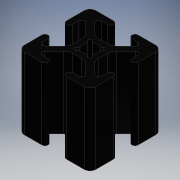
# Autodesk Inventor part: 1010-S-BLACK-FB
Saved by Autodesk Inventor 2017 SP1 (Build 210196100, 196)
## iProperties
Created: 2016-09-13
Part Number: 1010-S-BLACK-FB
Material: 6061-T6
Description: 40 S SHORT SINGLE UNIBEARING ASSEMBLY ON 40-4040 X 75mm
Document SubType Name: Modeling
Designer: BRALEF
Density: 1 g/cm^3
Appearance: BLACK ANODIZED
MATERIAL: 6061-T6
PART PRICE: 44.65
Author: BRALEF
Autodesk Inventor part; units mm, degrees
ref_plane "YZ Plane" through (0, 0, 0) normal (1, 0, 0) x (0, 1, 0)
ref_plane "XZ Plane" through (0, 0, 0) normal (0, 1, 0) x (-1, 0, 0)
ref_plane "XY Plane" through (0, 0, 0) normal (0, 0, 1) x (1, 0, 0)
sketch "Sketch1" plane through (0, 0, 0) normal (0, 1, 0) x (-1, 0, 0)
  arc A0 (-1.9692, 2.8605) -> (-2.8605, 1.9692) centre (-2.4696, 2.4696) ccw
  line L0 (-2.2319, 1.3405) -> (-2.8605, 1.9692)
  arc A1 (-2.2319, 1.3405) -> (-2.2319, -1.3405) centre (0, 0) ccw
  line L1 (-2.8605, -1.9692) -> (-2.2319, -1.3405)
  arc A2 (-2.8605, -1.9692) -> (-1.9692, -2.8605) centre (-2.4696, -2.4696) ccw
  line L2 (-1.3405, -2.2319) -> (-1.9692, -2.8605)
  arc A3 (-1.3405, -2.2319) -> (1.3405, -2.2319) centre (0, 0) ccw
  line L3 (1.9692, -2.8605) -> (1.3405, -2.2319)
  arc A4 (1.9692, -2.8605) -> (2.8605, -1.9692) centre (2.4696, -2.4696) ccw
  line L4 (2.2319, -1.3405) -> (2.8605, -1.9692)
  arc A5 (2.2319, -1.3405) -> (2.2319, 1.3405) centre (0, 0) ccw
  line L5 (2.8605, 1.9692) -> (2.2319, 1.3405)
  arc A6 (2.8605, 1.9692) -> (1.9692, 2.8605) centre (2.4696, 2.4696) ccw
  line L6 (1.3405, 2.2319) -> (1.9692, 2.8605)
  arc A7 (1.3405, 2.2319) -> (-1.3405, 2.2319) centre (0, 0) ccw
  line L7 (-1.9692, 2.8605) -> (-1.3405, 2.2319)
  arc A8 (-1.6396, -4.5172) -> (-3.8846, -5.4471) centre (-1.6396, -7.6922) ccw
  line L8 (-3.8846, -5.4471) -> (-7.1933, -8.7558)
  arc A9 (-7.1933, -8.7558) -> (-6.4749, -10.4902) centre (-6.4749, -9.4742) ccw
  line L9 (-6.4749, -10.4902) -> (-4.3561, -10.4902)
  arc A10 (-4.3561, -12.7) -> (-4.3561, -10.4902) centre (-4.3561, -11.5951) ccw
  line L10 (-4.3561, -12.7) -> (-10.5918, -12.7)
  arc A11 (-12.7, -10.5918) -> (-10.5918, -12.7) centre (-10.5918, -10.5918) ccw
  line L11 (-12.7, -10.5918) -> (-12.7, -4.3561)
  arc A12 (-10.4902, -4.3561) -> (-12.7, -4.3561) centre (-11.5951, -4.3561) ccw
  line L12 (-10.4902, -4.3561) -> (-10.4902, -6.4749)
  arc A13 (-10.4902, -6.4749) -> (-8.7558, -7.1933) centre (-9.4742, -6.4749) ccw
  line L13 (-8.7558, -7.1933) -> (-5.4471, -3.8846)
  arc A14 (-5.4471, -3.8846) -> (-4.5172, -1.6396) centre (-7.6922, -1.6396) ccw
  line L14 (-4.5172, -1.6396) -> (-4.5172, 1.6396)
  arc A15 (-4.5172, 1.6396) -> (-5.4471, 3.8846) centre (-7.6922, 1.6396) ccw
  line L15 (-5.4471, 3.8846) -> (-8.7558, 7.1933)
  arc A16 (-8.7558, 7.1933) -> (-10.4902, 6.4749) centre (-9.4742, 6.4749) ccw
  line L16 (-10.4902, 6.4749) -> (-10.4902, 4.3561)
  arc A17 (-12.7, 4.3561) -> (-10.4902, 4.3561) centre (-11.5951, 4.3561) ccw
  line L17 (-12.7, 4.3561) -> (-12.7, 10.5918)
  arc A18 (-10.5918, 12.7) -> (-12.7, 10.5918) centre (-10.5918, 10.5918) ccw
  line L18 (-10.5918, 12.7) -> (-4.3561, 12.7)
  arc A19 (-4.3561, 10.4902) -> (-4.3561, 12.7) centre (-4.3561, 11.5951) ccw
  line L19 (-4.3561, 10.4902) -> (-6.4749, 10.4902)
  arc A20 (-6.4749, 10.4902) -> (-7.1933, 8.7558) centre (-6.4749, 9.4742) ccw
  line L20 (-7.1933, 8.7558) -> (-3.8846, 5.4471)
  arc A21 (-3.8846, 5.4471) -> (-1.6396, 4.5172) centre (-1.6396, 7.6922) ccw
  line L21 (-1.6396, 4.5172) -> (1.6396, 4.5172)
  arc A22 (1.6396, 4.5172) -> (3.8846, 5.4471) centre (1.6396, 7.6922) ccw
  line L22 (3.8846, 5.4471) -> (7.1933, 8.7558)
  arc A23 (7.1933, 8.7558) -> (6.4749, 10.4902) centre (6.4749, 9.4742) ccw
  line L23 (6.4749, 10.4902) -> (4.3561, 10.4902)
  arc A24 (4.3561, 12.7) -> (4.3561, 10.4902) centre (4.3561, 11.5951) ccw
  line L24 (4.3561, 12.7) -> (10.5918, 12.7)
  arc A25 (12.7, 10.5918) -> (10.5918, 12.7) centre (10.5918, 10.5918) ccw
  line L25 (12.7, 10.5918) -> (12.7, 4.3561)
  arc A26 (10.4902, 4.3561) -> (12.7, 4.3561) centre (11.5951, 4.3561) ccw
  line L26 (10.4902, 4.3561) -> (10.4902, 6.4749)
  arc A27 (10.4902, 6.4749) -> (8.7558, 7.1933) centre (9.4742, 6.4749) ccw
  line L27 (8.7558, 7.1933) -> (5.4471, 3.8846)
  arc A28 (5.4471, 3.8846) -> (4.5172, 1.6396) centre (7.6922, 1.6396) ccw
  line L28 (4.5172, 1.6396) -> (4.5172, -1.6396)
  arc A29 (4.5172, -1.6396) -> (5.4471, -3.8846) centre (7.6922, -1.6396) ccw
  line L29 (5.4471, -3.8846) -> (8.7558, -7.1933)
  arc A30 (8.7558, -7.1933) -> (10.4902, -6.4749) centre (9.4742, -6.4749) ccw
  line L30 (10.4902, -6.4749) -> (10.4902, -4.3561)
  arc A31 (12.7, -4.3561) -> (10.4902, -4.3561) centre (11.5951, -4.3561) ccw
  line L31 (12.7, -4.3561) -> (12.7, -10.5918)
  arc A32 (10.5918, -12.7) -> (12.7, -10.5918) centre (10.5918, -10.5918) ccw
  line L32 (10.5918, -12.7) -> (4.3561, -12.7)
  arc A33 (4.3561, -10.4902) -> (4.3561, -12.7) centre (4.3561, -11.5951) ccw
  line L33 (4.3561, -10.4902) -> (6.4749, -10.4902)
  arc A34 (6.4749, -10.4902) -> (7.1933, -8.7558) centre (6.4749, -9.4742) ccw
  line L34 (7.1933, -8.7558) -> (3.8846, -5.4471)
  arc A35 (3.8846, -5.4471) -> (1.6396, -4.5172) centre (1.6396, -7.6922) ccw
  line L35 (1.6396, -4.5172) -> (-1.6396, -4.5172)
  dimension "d0" = 1.1049
  dimension "d1" = 2.1082
  dimension "d2" = 1.016
  dimension "d3" = 3.175
  dimension "d4" = 0.635
  dimension "d5" = 2.6035
  dimension "d6" = 2.6035
  dimension "d7" = 2.6035
  dimension "d8" = 2.6035
  dimension "d9" = 45
  dimension "d10" = 45
  dimension "d11" = 45
  dimension "d12" = 45
  dimension "d13" = 45
  dimension "d14" = 45
  dimension "d15" = 45
  dimension "d16" = 90
  dimension "d17" = 90
  dimension "d18" = 45
  dimension "d19" = 45
  dimension "d20" = 90
  dimension "d21" = 90
  dimension "d22" = 90
  dimension "d23" = 90
  dimension "d24" = 90
  dimension "d25" = 90
  dimension "d26" = 8.1828
  dimension "d27" = 17.2172
  dimension "d28" = 23.1902
  dimension "d29" = 25.4
  dimension "d30" = 8.1828
  dimension "d31" = 17.2172
  dimension "d32" = 2.2096
  dimension "d33" = 0.4746
  dimension "d34" = 1.7351
  dimension "d35" = 1.2605
  dimension "d36" = 0.4746
  dimension "d37" = 1.7351
  dimension "d38" = 12.7
  dimension "d39" = 12.7
  dimension "d40" = 10.4902
  dimension "d41" = 12.7
  dimension "d42" = 1.1048
  dimension "d43" = 1.1048
  dimension "d44" = 1.1048
  dimension "d45" = 0.6303
  dimension "d46" = 0.6303
  dimension "d47" = 0.6303
  dimension "d48" = 0.6303
  dimension "d49" = 0.6303
  dimension "d50" = 10.4902
  dimension "d51" = 10.4902
  dimension "d52" = 1.1048
  dimension "d53" = 1.1048
  dimension "d54" = 12.7
  dimension "d55" = 12.7
  dimension "d56" = 10.4902
  dimension "d57" = 12.7
  dimension "d58" = 8.3439
  dimension "d59" = 17.0561
  dimension "d60" = 8.3439
  dimension "d61" = 8.3439
  dimension "d62" = 9.8395
  dimension "d63" = 9.8395
  constraints: 72 end point, 72 point on circle, 56 tangent, 36 centre point, 23 equal radius, 16 parallel, 1 horizontal, 1 perpendicular, 1 vertical
  measures "d0" radius of A26
  measures "d1" radius of A25
  measures "d2" radius of A27
  measures "d3" radius of A28
  measures "d4" radius of A6
  measures "d5" radius of A7
  measures "d6" radius of A1
  measures "d7" radius of A5
  measures "d8" radius of A3
  measures "d9" angle of L25 L27
  measures "d10" angle of L25 L29
  measures "d11" angle of L25 L34
  measures "d12" angle of L25 L5
  measures "d13" angle of L25 L6
  measures "d14" angle of L25 L7
  measures "d15" angle of L25 L0
  measures "d16" angle of L25 L19
  measures "d17" angle of L25 L9
  measures "d18" angle of L25 L8
  measures "d19" angle of L25 L13
  measures "d20" angle of L25 L18
  measures "d21" angle of L25 L10
  measures "d22" angle of L31 L24
  measures "d23" angle of L30 L24
  measures "d24" angle of L24 L12
  measures "d25" angle of L24 L11
  measures "d26" distance between parallel lines of L25 L28
  measures "d27" distance between parallel lines of L25 L14
  measures "d28" distance between parallel lines of L25 L16
  measures "d29" distance between parallel lines of L24 L32
  measures "d30" distance between parallel lines of L24 L21
  measures "d31" distance between parallel lines of L24 L35
  measures "d32" distance between parallel lines of L27 L22
  measures "d33" distance between parallel lines of L2 L27
  measures "d34" distance between parallel lines of L1 L27
  measures "d35" distance between parallel lines of L4 L3
  measures "d36" distance between parallel lines of L4 L20
  measures "d37" distance between parallel lines of L4 L15
  measures "d38" distance from line of point (0, 0) L25
  measures "d39" distance from line of point (0, 0) L31
  measures "d40" distance from line of point (0, 0) L30
  measures "d41" distance from line of point (0, 0) L24
  measures "d42" distance from line of point (0, 0) L27
  measures "d43" distance from line of point (0, 0) L29
  measures "d44" distance from line of point (0, 0) L34
  measures "d45" distance from line of point (0, 0) L5
  measures "d46" distance from line of point (0, 0) L4
  measures "d47" distance from line of point (0, 0) L6
  measures "d48" distance from line of point (0, 0) L7
  measures "d49" distance from line of point (0, 0) L0
  measures "d50" distance from line of point (0, 0) L19
  measures "d51" distance from line of point (0, 0) L9
  measures "d52" distance from line of point (0, 0) L8
  measures "d53" distance from line of point (0, 0) L13
  measures "d54" distance from line of point (0, 0) L18
  measures "d55" distance from line of point (0, 0) L10
  measures "d56" distance from line of point (0, 0) L12
  measures "d57" distance from line of point (0, 0) L11
  measures "d58" distance from line of L25.end L24
  measures "d59" distance from line of L31.start L24
  measures "d60" distance from line of L24.start L25
  measures "d61" distance from line of L33.start L25
  measures "d62" distance from line of L5.start L25
  measures "d63" distance from line of L4.end L25
extrude "Extrusion1" add sketch "Sketch1" along normal mid plane 25.4
body "Solid1"
